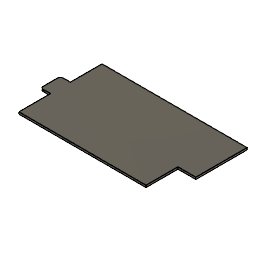
Control board - middle low plate v4 (Autodesk Fusion 360 design; units mm, degrees)
Autodesk Fusion 360 part; units mm, degrees
sketch "Sketch1" plane through (0, 0, 0) normal (0, 0, 1) x (1, 0, 0)
  line L0 (3.6667, 44.4476) -> (76.5667, 44.4476)
  line L1 (76.5667, 44.4476) -> (76.5667, 2.6476)
  line L2 (76.5667, 2.6476) -> (3.6667, 2.6476)
  line L3 (3.6667, 2.6476) -> (3.6667, 44.4476)
  line L4 (3.6667, 23.5476) -> (76.5667, 23.5476) construction
  line L5 (3.6667, 28.5476) -> (-0.0333, 28.5476)
  line L6 (-1.3333, 27.2476) -> (-1.3333, 19.8476)
  line L7 (-0.0333, 18.5476) -> (3.6667, 18.5476)
  line L8 (3.6667, 18.5476) -> (3.6667, 28.5476)
  arc A0 (-0.0333, 28.5476) -> (-1.3333, 27.2476) centre (-0.0333, 27.2476) ccw
  arc A1 (-1.3333, 19.8476) -> (-0.0333, 18.5476) centre (-0.0333, 19.8476) ccw
  line L9 (76.5667, 2.6476) -> (67.5667, 2.6476)
  line L10 (67.5667, 2.6476) -> (67.5667, 18.6476)
  line L11 (67.5667, 18.6476) -> (76.5667, 18.6476)
  line L12 (76.5667, 18.6476) -> (76.5667, 2.6476)
  point P0 (-1.3333, 28.5476)
  point P1 (-1.3333, 18.5476)
  dimension "d1" = 72.9
  dimension "d2" = 41.8
  dimension "d7" = 10
  dimension "d8" = 5
  dimension "d9" = 1.3
  dimension "d10" = 16
  dimension "d11" = 9
  constraint horizontal L0
  constraint vertical L1
  constraint horizontal L2
  constraint vertical L3
  constraint midpoint L3 L4.start
  constraint midpoint L1 L4.end
  constraint horizontal L5
  constraint vertical L6
  constraint horizontal L7
  constraint vertical L8
  constraint coincident L3 L5.start
  constraint symmetric L4 L5 L7
  constraint coincident P0 L5
  constraint coincident P0 L6
  constraint tangent L5 A0
  constraint tangent L6 A0
  constraint coincident P1 L6
  constraint coincident P1 L7
  constraint tangent L6 A1
  constraint tangent L7 A1
  constraint equal A0 A1
  constraint horizontal L9
  constraint vertical L10
  constraint horizontal L11
  constraint vertical L12
  measures "d1" distance of L0.start L0.end
  measures "d2" distance of L0.end L1.end
  measures "d7" distance of P0 P1
  measures "d8" distance of L5.start P0
  measures "d9" radius of A0
  measures "d10" distance of L9.end L10.end
  measures "d11" distance of L10.end L11.end
extrude "Extrude1" add sketch "Sketch1" along normal blind 1 contours L0 L1 L2 L3 L8 L10 L11 | L3 L5 L6 L7 L8 A0 A1
